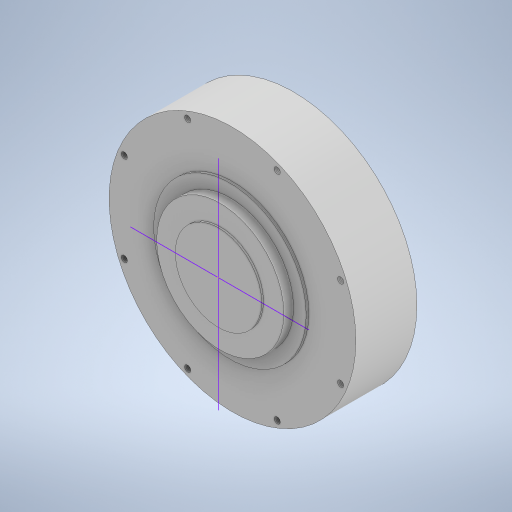
# Autodesk Inventor part: GIM8108-8
Saved by Autodesk Inventor 2023 (Build 270158000, 158)
## iProperties
Created: 2024-10-18
Part Number: GIM8108-8
Material: 一般
Document SubType Name: Modeling
Designer: 佐藤智貴
Density: 1 g/cm^3
Appearance: 既定
Author: 佐藤智貴
Autodesk Inventor part; units mm, degrees
ref_plane "YZ Plane" through (0, 0, 0) normal (1, 0, 0) x (0, 1, 0)
ref_plane "XZ Plane" through (0, 0, 0) normal (0, 1, 0) x (-1, 0, 0)
ref_plane "XY Plane" through (0, 0, 0) normal (0, 0, 1) x (1, 0, 0)
sketch "スケッチ1" plane through (0, 0, 0) normal (0, 0, 1) x (1, 0, 0)
  circle A0 centre (0, 0) radius 46
  line L0 (0, 54.251) -> (0, -59.4354)
  line L1 (-57.6108, 0) -> (60.5194, 0)
  circle A1 centre (0, 0) radius 48.5
  line L2 (0, 0) -> (-23.2819, 56.2075)
  line L3 (-23.2819, 56.2075) -> (0, 0)
  line L4 (0, 0) -> (23.2706, 56.1801)
  point P0 (-17.6034, 42.4985)
  point P1 (17.6034, 42.4985)
  point P2 (-42.4985, -17.6034)
  point P3 (-42.4985, 17.6034)
  point P4 (17.6034, -42.4985)
  point P5 (-17.6034, -42.4985)
  point P6 (42.4985, 17.6034)
  point P7 (42.4985, -17.6034)
  dimension "d0" = 92
  dimension "d1" = 97
  dimension "d2" = 45
  dimension "d3" = 22.5
  dimension "d6" = 360
  constraints: 10 end point, 2 centre point, 2 coincident, 2 point on circle, 2 point on line, 1 collinear, 1 horizontal, 1 vertical, 9 other
  measures "d0" diameter of A0
  measures "d1" diameter of A1
  measures "d2" angle of L4 L2
  measures "d3" angle of L2 L0
extrude "押し出し1" add sketch "スケッチ1" along normal blind 24
sketch "スケッチ2" plane through (0, 0, 24) normal (0, 0, 1) x (1, 0, 0)
  line L0 (0, 68.9903) -> (0, -65.3185)
  circle A0 centre (0, 0) radius 46
  line L1 (0, 0) -> (-21.3879, 51.6351)
  line L2 (-21.3879, 51.6351) -> (0, 0)
  line L3 (0, 0) -> (19.8653, 47.959)
  point P0 (-17.6034, 42.4985)
  point P1 (17.6034, 42.4985)
  point P2 (-42.4985, -17.6034)
  point P3 (-42.4985, 17.6034)
  point P4 (17.6034, -42.4985)
  point P5 (-17.6034, -42.4985)
  point P6 (42.4985, 17.6034)
  point P7 (42.4985, -17.6034)
  dimension "d10" = 92
  dimension "d11" = 45
  dimension "d12" = 22.5
  dimension "d15" = 360
  constraints: 8 end point, 2 point on circle, 2 point on line, 1 centre point, 1 coincident, 1 collinear, 1 vertical, 9 other
  measures "d10" diameter of A0
  measures "d11" angle of L3 L1
  measures "d12" angle of L1 L0
hole "穴1" at (-17.6034, 42.4985, 24) at (17.6034, 42.4985, 24) at (-42.4985, -17.6034, 24) at (-42.4985, 17.6034, 24) at (17.6034, -42.4985, 24) at (-17.6034, -42.4985, 24) at (42.4985, 17.6034, 24) at (42.4985, -17.6034, 24) direction (0, 0, -1) diameter 2.459 end through all thread size "M3x0.5" class "6H" standard "ISO Metric profile"
sketch "スケッチ3" plane through (0, 0, 24) normal (0, 0, 1) x (1, 0, 0)
  circle A0 centre (0, 0) radius 30
  dimension "d24" = 60
  constraints: 1 centre point, 1 coincident
  measures "d24" diameter of A0
extrude "押し出し2" add sketch "スケッチ3" along normal blind 1
sketch "スケッチ4" plane through (0, 0, 25) normal (0, 0, 1) x (1, 0, 0)
  circle A0 centre (0, 0) radius 25
  dimension "d27" = 50
  constraints: 1 centre point, 1 coincident
  measures "d27" diameter of A0
extrude "押し出し3" add sketch "スケッチ4" along normal blind 3.8
sketch "スケッチ5" plane through (0, 0, 28.8) normal (0, 0, 1) x (1, 0, 0)
  circle A0 centre (0, 0) radius 17
  dimension "d30" = 34
  constraints: 1 centre point, 1 coincident
  measures "d30" diameter of A0
extrude "押し出し4" add sketch "スケッチ5" along normal blind 0.7
sketch "スケッチ6" plane through (0, 0, 29.5) normal (0, 0, 1) x (1, 0, 0)
  line L0 (0, 40.5289) -> (0, -45.0936)
  line L1 (-34.581, 0) -> (35.411, 0)
  point P0 (0, 0)
  constraints: 4 end point, 1 horizontal, 1 vertical
